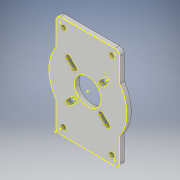
# Autodesk Inventor part: TapaSuperior
Saved by Autodesk Inventor 2019 (Build 230136000, 136)
## iProperties
Created: 2019-03-04
Part Number: TapaSuperior
Material: Generic
Document SubType Name: Modeling
Designer: Kenny
Density: 1 g/cm^3
Appearance: Default
Author: Kenny
Autodesk Inventor part; units mm, degrees
ref_plane "YZ Plane" through (0, 0, 0) normal (1, 0, 0) x (0, 1, 0)
ref_plane "XZ Plane" through (0, 0, 0) normal (0, 1, 0) x (-1, 0, 0)
ref_plane "XY Plane" through (0, 0, 0) normal (0, 0, 1) x (1, 0, 0)
sketch "Sketch1" plane through (0, 0, 0) normal (0, 0, 1) x (1, 0, 0)
  line L0 (0, 0) -> (41, 0) construction
  line L1 (41, 0) -> (41, 65.3) construction
  line L2 (41, 65.3) -> (0, 65.3) construction
  circle A0 centre (20.5, 32.65) radius 8.5
  line L3 (0, 0) -> (41, 0)
  line L4 (41, 65.3) -> (0, 65.3)
  line L5 (20.5, 65.3) -> (20.5, 0) construction
  line L6 (0, 32.65) -> (41, 32.65) construction
  line L7 (0, 65.3) -> (0, 46.9591) construction
  line L8 (0, 18.3409) -> (0, 0) construction
  line L9 (0, 65.3) -> (0, 46.9591)
  line L10 (0, 18.3409) -> (0, 0)
  line L11 (41, 0) -> (41, 18.3409)
  line L12 (41, 46.9591) -> (41, 65.3)
  arc A1 (0, 46.9591) -> (0, 18.3409) centre (20.5, 32.65) ccw
  arc A2 (41, 18.3409) -> (41, 46.9591) centre (20.5, 32.65) ccw
  point P0 (5, 60.3)
  point P1 (36, 60.3)
  point P2 (5, 5)
  point P3 (36, 5)
  point P4 (12, 41.15)
  point P5 (8, 45.15)
  point P6 (29, 41.15)
  point P7 (33, 45.15)
  point P8 (29, 24.15)
  point P9 (12, 24.15)
  point P10 (8, 20.15)
  point P11 (33, 20.15)
  dimension "d3" = 17
  dimension "d5" = 5
  dimension "d6" = 5
  dimension "d7" = 5
  dimension "d10" = 12.5
  dimension "d11" = 25
  dimension "d12" = 25
  dimension "d13" = 17
  dimension "d14" = 17
  dimension "d15" = 8.5
  dimension "d16" = 24.15
  dimension "d17" = 20.15
  dimension "d18" = 32.65
  dimension "d20" = 41
  dimension "d22" = 65.3
  dimension "d23" = 5
  dimension "d25" = 41
  dimension "d26" = 5
  dimension "d27" = 16.5
  constraints: 26 end point, 8 parallel, 6 horizontal alignment, 6 vertical alignment, 4 point on circle, 3 centre point, 3 perpendicular, 2 horizontal, 2 midpoint, 1 coincident
  measures "d3" diameter of A0
  measures "d5" distance from line of point (5, 60.3) L2
  measures "d6" distance from line of L1 point (36, 5)
  measures "d7" distance from line of L0 point (36, 5)
  measures "d10" distance from line of L5 point (33, 45.15)
  measures "d11" distance of point (33, 45.15) point (8, 45.15)
  measures "d12" distance of point (8, 20.15) point (8, 45.15)
  measures "d13" distance of point (29, 24.15) point (12, 24.15)
  measures "d14" distance of point (29, 24.15) point (29, 41.15)
  measures "d15" distance from line of L5 point (12, 41.15)
  measures "d16" distance from line of L0 point (12, 24.15)
  measures "d17" distance from line of L0 point (8, 20.15)
  measures "d18" distance from line of L0 A1.centre
  measures "d20" distance between parallel lines of L8 L11
  measures "d22" distance between parallel lines of L0 L2
  measures "d23" distance from line of L7 point (5, 60.3)
  measures "d25" distance between parallel lines of L1 L7
  measures "d26" distance from line of L10 point (5, 5)
  measures "d27" radial gap between concentric circles of A0 A2
extrude "Extrusion1" add sketch "Sketch1" along normal blind 3
sketch "Sketch2" plane through (0, 0, 0) normal (0, 0, 1) x (1, 0, 0)
  line L0 (0, 0) -> (41, 0) construction
  line L1 (41, 0) -> (41, 65.3) construction
  line L2 (41, 65.3) -> (0, 65.3) construction
  circle A0 centre (20.5, 32.65) radius 8.5
  line L3 (0, 0) -> (41, 0)
  line L4 (41, 65.3) -> (0, 65.3)
  line L5 (20.5, 65.3) -> (20.5, 0) construction
  line L6 (0, 32.65) -> (41, 32.65) construction
  line L7 (0, 65.3) -> (0, 46.9591) construction
  line L8 (0, 18.3409) -> (0, 0) construction
  line L9 (0, 65.3) -> (0, 46.9591)
  line L10 (0, 18.3409) -> (0, 0)
  line L11 (41, 0) -> (41, 18.3409)
  line L12 (41, 46.9591) -> (41, 65.3)
  arc A1 (0, 46.9591) -> (0, 18.3409) centre (20.5, 32.65) ccw
  arc A2 (41, 18.3409) -> (41, 46.9591) centre (20.5, 32.65) ccw
  point P0 (5, 60.3)
  point P1 (36, 60.3)
  point P2 (5, 5)
  point P3 (36, 5)
  point P4 (12, 41.15)
  point P5 (8, 45.15)
  point P6 (29, 41.15)
  point P7 (33, 45.15)
  point P8 (29, 24.15)
  point P9 (12, 24.15)
  point P10 (8, 20.15)
  point P11 (33, 20.15)
  dimension "d30" = 17
  dimension "d31" = 5
  dimension "d32" = 5
  dimension "d33" = 5
  dimension "d34" = 12.5
  dimension "d35" = 25
  dimension "d36" = 25
  dimension "d37" = 17
  dimension "d38" = 17
  dimension "d39" = 8.5
  dimension "d40" = 24.15
  dimension "d41" = 20.15
  dimension "d42" = 32.65
  dimension "d43" = 41
  dimension "d44" = 65.3
  dimension "d45" = 5
  dimension "d46" = 41
  dimension "d47" = 5
  dimension "d48" = 16.5
  constraints: 26 end point, 8 parallel, 6 horizontal alignment, 6 vertical alignment, 4 point on circle, 3 centre point, 3 perpendicular, 2 horizontal, 2 midpoint, 1 coincident
  measures "d30" diameter of A0
  measures "d31" distance from line of point (5, 60.3) L2
  measures "d32" distance from line of L1 point (36, 5)
  measures "d33" distance from line of L0 point (36, 5)
  measures "d34" distance from line of L5 point (33, 45.15)
  measures "d35" distance of point (33, 45.15) point (8, 45.15)
  measures "d36" distance of point (8, 20.15) point (8, 45.15)
  measures "d37" distance of point (29, 24.15) point (12, 24.15)
  measures "d38" distance of point (29, 24.15) point (29, 41.15)
  measures "d39" distance from line of L5 point (12, 41.15)
  measures "d40" distance from line of L0 point (12, 24.15)
  measures "d41" distance from line of L0 point (8, 20.15)
  measures "d42" distance from line of L0 A1.centre
  measures "d43" distance between parallel lines of L8 L11
  measures "d44" distance between parallel lines of L0 L2
  measures "d45" distance from line of L7 point (5, 60.3)
  measures "d46" distance between parallel lines of L1 L7
  measures "d47" distance from line of L10 point (5, 5)
  measures "d48" radial gap between concentric circles of A0 A2
hole "Hole1" at (5, 60.3, 0) at (36, 60.3, 0) at (5, 5, 0) at (36, 5, 0) at (12, 41.15, 0) at (8, 45.15, 0) at (29, 41.15, 0) at (33, 45.15, 0) at (29, 24.15, 0) at (12, 24.15, 0) at (8, 20.15, 0) at (33, 20.15, 0) direction (0, 0, 1) diameter 3.3 end through all
sketch "Sketch3" plane through (0, 0, 3) normal (0, 0, 1) x (1, 0, 0)
  circle A0 centre (8, 45.15) radius 1.65 projected
  line L0 (9.1667, 46.3167) -> (13.1667, 42.3167)
  circle A1 centre (12, 41.15) radius 1.65 projected
  circle A2 centre (33, 20.15) radius 1.65 projected
  circle A3 centre (29, 24.15) radius 1.65 projected
  circle A4 centre (33, 20.15) radius 1.65 projected
  circle A5 centre (29, 24.15) radius 1.65 projected
  line L1 (10.8333, 39.9833) -> (6.8333, 43.9833)
  circle A6 centre (33, 45.15) radius 1.65 projected
  circle A7 centre (29, 41.15) radius 1.65 projected
  circle A8 centre (33, 45.15) radius 1.65 projected
  circle A9 centre (8, 20.15) radius 1.65 projected
  line L2 (6.8333, 21.3167) -> (10.8333, 25.3167)
  line L3 (13.1667, 22.9833) -> (9.1667, 18.9833)
  circle A10 centre (12, 24.15) radius 1.65 projected
  line L4 (27.8333, 42.3167) -> (31.8333, 46.3167)
  line L5 (30.1667, 39.9833) -> (34.1667, 43.9833)
  line L6 (27.8333, 22.9833) -> (31.8333, 18.9833)
  line L7 (34.1667, 21.3167) -> (30.1667, 25.3167)
  point P0 (0, 0)
  constraints: 17 tangent, 16 end point, 14 point on circle
extrude "Extrusion2" cut sketch "Sketch3" against normal blind 3 contours A0 L0 A1 L1 | A2 L6 A3 L7 | A6 L5 A7 L4 | A9 L2 A10 L3
fillet "Fillet1" radius 3 4 edges at (41, 65.3, 1.5) (0, 65.3, 1.5) (0, 0, 1.5) (41, 0, 1.5)
sketch "Sketch4" plane through (0, 0, 3) normal (0, 0, 1) x (1, 0, 0)
  line L0 (13.1667, 22.9833) -> (9.1667, 18.9833) projected
  arc A0 (6.8333, 21.3167) -> (9.1667, 18.9833) centre (8, 20.15) ccw projected
  line L1 (6.8333, 21.3167) -> (10.8333, 25.3167) projected
  arc A1 (13.1667, 22.9833) -> (10.8333, 25.3167) centre (12, 24.15) ccw projected
  line L2 (31.8333, 18.9833) -> (27.8333, 22.9833) projected
  arc A2 (30.1667, 25.3167) -> (27.8333, 22.9833) centre (29, 24.15) ccw projected
  line L3 (30.1667, 25.3167) -> (34.1667, 21.3167) projected
  arc A3 (31.8333, 18.9833) -> (34.1667, 21.3167) centre (33, 20.15) ccw projected
  line L4 (34.1667, 43.9833) -> (30.1667, 39.9833) projected
  arc A4 (27.8333, 42.3167) -> (30.1667, 39.9833) centre (29, 41.15) ccw projected
  line L5 (27.8333, 42.3167) -> (31.8333, 46.3167) projected
  arc A5 (34.1667, 43.9833) -> (31.8333, 46.3167) centre (33, 45.15) ccw projected
  circle A6 centre (5, 5) radius 1.65 projected
  circle A7 centre (5, 60.3) radius 1.65 projected
  circle A8 centre (36, 60.3) radius 1.65 projected
  circle A9 centre (36, 5) radius 1.65 projected
  line L6 (10.8333, 39.9833) -> (6.8333, 43.9833) projected
  arc A10 (9.1667, 46.3167) -> (6.8333, 43.9833) centre (8, 45.15) ccw projected
  line L7 (9.1667, 46.3167) -> (13.1667, 42.3167) projected
  arc A11 (10.8333, 39.9833) -> (13.1667, 42.3167) centre (12, 41.15) ccw projected
  circle A12 centre (20.5, 32.65) radius 8.5 projected
  arc A13 (38, 0) -> (41, 3) centre (38, 3) ccw projected
  line L8 (41, 3) -> (41, 18.3409) projected
  arc A14 (41, 18.3409) -> (41, 46.9591) centre (20.5, 32.65) ccw projected
  line L9 (41, 46.9591) -> (41, 62.3) projected
  arc A15 (41, 62.3) -> (38, 65.3) centre (38, 62.3) ccw projected
  line L10 (38, 65.3) -> (3, 65.3) projected
  arc A16 (3, 65.3) -> (0, 62.3) centre (3, 62.3) ccw projected
  line L11 (0, 62.3) -> (0, 46.9591) projected
  arc A17 (0, 46.9591) -> (0, 18.3409) centre (20.5, 32.65) ccw projected
  line L12 (0, 18.3409) -> (0, 3) projected
  arc A18 (0, 3) -> (3, 0) centre (3, 3) ccw projected
  line L13 (3, 0) -> (38, 0) projected
  point P0 (0, 0)
body "Solid1"
